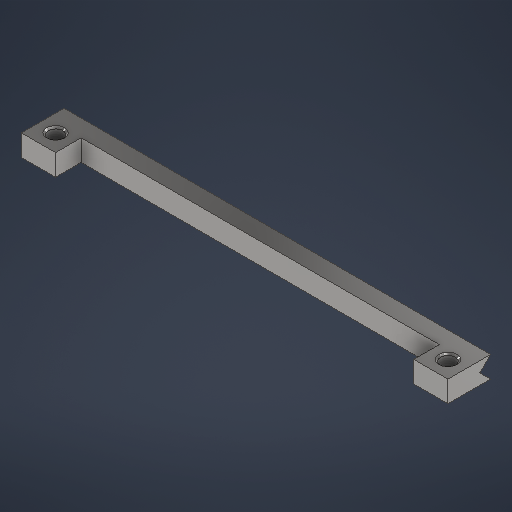
# Autodesk Inventor part: K-tor-kulek-blatu
Saved by Autodesk Inventor 2026.1 (Build 301233020, 233B)
## iProperties
Created: 2025-11-03
Part Number: K-tor-kulek-blatu
Material: Steel, High Strength, Low Alloy
Document SubType Name: Modeling
Designer: Jan
Density: 7.85 g/cm^3
Appearance: Steel - Polished
Author: Jan
Autodesk Inventor part; units mm, degrees
ref_plane "YZ Plane" through (0, 0, 0) normal (1, 0, 0) x (0, 1, 0)
ref_plane "XZ Plane" through (0, 0, 0) normal (0, 1, 0) x (-1, 0, 0)
ref_plane "XY Plane" through (0, 0, 0) normal (0, 0, 1) x (1, 0, 0)
sketch "Sketch1" plane through (0, 0, 0) normal (1, 0, 0) x (0, 1, 0)
  line L0 (0, 0) -> (5, 0)
  line L1 (5, 0) -> (5, -10)
  line L2 (5, -10) -> (2.5, -7.5)
  line L3 (2.5, -7.5) -> (0, -10)
  line L4 (0, 0) -> (0, -10)
  line L5 (2.5, -7.5) -> (2.5, -12.5) construction
  circle A0 centre (2.5, -10.3284) radius 2 construction
  line L6 (2.5, -10.3284) -> (1.25, -10.3284) construction
  line L7 (5, -10.6569) -> (2.5, -13.1569) construction
  line L8 (2.5, -13.1569) -> (0, -10.6569) construction
  dimension "d0" = 5
  dimension "d3" = 10
  dimension "d4" = 4
  dimension "d33" = 0.6569
  dimension "d34" = 5.6569
  dimension "d35" = 2.8284
  constraints: 18 end point, 3 symmetric about line, 2 horizontal, 2 perpendicular, 2 vertical, 1 centre point, 1 horizontal alignment, 1 parallel, 1 point on line, 1 tangent
  measures "d0" distance of L0.start L0.end
  measures "d3" distance of L0.end L1.end
  measures "d4" diameter of A0
  measures "d33" distance of L7.start L1.end
  measures "d34" distance of L8.start L2.end
  measures "d35" distance of L8.start L6.start
extrude "Extrusion1" add sketch "Sketch1" along normal blind 100
sketch "Sketch2" plane through (0, 5, 0) normal (0, 1, 0) x (1, 0, 0)
  line L0 (0, 10) -> (0, 0) construction
  line L1 (0, 0) -> (100, 0) construction
  line L2 (0, 10) -> (100, 10) construction
  line L3 (4, 0) -> (4, 10) construction
  line L4 (50, 0) -> (50, 15) construction
  circle A0 centre (4, 4) radius 2
  circle A1 centre (96, 4) radius 2
  point P0 (0, 5)
  dimension "d8" = 10
  dimension "d10" = 4
  dimension "d12" = 15
  dimension "d13" = 50
  dimension "d14" = 4
  dimension "d15" = 4
  constraints: 4 end point, 3 point on line, 2 centre point, 2 midpoint, 1 perpendicular, 1 symmetric about line, 1 vertical, 1 other
  measures "d8" distance between parallel lines of L2 L1
  measures "d10" distance from line of L0.end L3
  measures "d12" distance of L4.start L4.end
  measures "d13" distance from line of L0.start L4
  measures "d14" diameter of A0
  measures "d15" horizontal distance of L0.end A0.centre
hole "Hole1" at (4, 5, -4) direction (0, -1, 0) diameter 3.4587 end through all thread size "M4x0.5" class "6H" standard "ISO Metric profile"
hole "Hole2" at (96, 5, -4) direction (0, -1, 0) diameter 3.4587 end through all thread size "M4x0.5" class "6H" standard "ISO Metric profile"
chamfer "Chamfer2" distance 0.4 angle 45 2 edges at (4, 5, -5.7294) (96, 5, -5.7294)
sketch "Sketch3" plane through (0, 0, 0) normal (0, 0, 1) x (1, 0, 0)
  line L0 (0, 5) -> (100, 5) projected
  line L1 (0, 0) -> (100, 0) projected
  line L2 (8, 5) -> (92, 5)
  line L3 (92, 5) -> (92, 0)
  line L4 (92, 0) -> (8, 0)
  line L5 (8, 0) -> (8, 5)
  line L6 (0, 5) -> (0, 0) projected
  point P0 (0, 2.5)
  point P1 (8, 0)
  point P2 (92, 5)
  dimension "d39" = 84
  dimension "d40" = 8
  constraints: 8 end point, 2 parallel, 2 point on line, 1 horizontal, 1 midpoint, 1 perpendicular
  measures "d39" distance of L3.end L4.end
  measures "d40" distance from line of point (0, 2.5) L5
extrude "Extrusion2" cut sketch "Sketch3" against normal blind 6 contours L0 L3 L1 L5
body "Solid1"
